GearboxTop_v3 (Autodesk Fusion 360 design; units mm, degrees)
Autodesk Fusion 360 part; units mm, degrees
sketch "Sketch1" plane through (0, 0, 0) normal (0, 0, 1) x (1, 0, 0)
  circle A0 centre (0, 0) radius 65
  circle A1 centre (0, 0) radius 61.0225 construction
  circle A2 centre (0, 0) radius 39.5
  circle A3 centre (0, -61.0225) radius 1.5
  dimension "d1" = 130
  dimension "d2" = 122.045
  dimension "d3" = 79
  dimension "ScrewDia" = 3
  constraint coincident A0.centre A1.centre
  constraint concentric A0 A1
  constraint coincident A1 A3.centre
  measures "d1" diameter of A0
  measures "d2" diameter of A1
  measures "d3" diameter of A2
  measures "ScrewDia" diameter of A3
extrude "Extrude1" add sketch "Sketch1" along normal blind 2 contours A0 | A3
sketch "Sketch2" plane through (0, 0, 2) normal (0, 0, 1) x (-1, 0, 0)
  circle A0 centre (0, 0) radius 39.5
  circle A1 centre (0, 0) radius 65
  circle A2 centre (0, 0) radius 42.5
  dimension "BearingDia" = 85
  constraint coincident A0.centre A1.centre
  measures "BearingDia" diameter of A2
extrude "Extrude2" add sketch "Sketch2" along normal blind 10 contours A1
extrude "Extrude3" cut sketch "Sketch1" along normal blind 25 contours A3
sketch "Sketch3" plane through (0, 0, 12) normal (0, 0, 1) x (-1, 0, 0)
  circle A0 centre (0, 61.0225) radius 1.5
  circle A1 centre (0, 0) radius 42.5
  circle A2 centre (0, 0) radius 65
  circle A3 centre (0, -61.0225) radius 2.5
  dimension "ScrewHeadDia" = 5
  measures "ScrewHeadDia" diameter of A3
extrude "Extrude4" cut sketch "Sketch3" against normal blind 3 contours A3
sketch "Sketch6" plane through (0, 0, 0) normal (0, 0, -1) x (1, 0, 0)
  circle A0 centre (0, 61.0225) radius 1.5
  circle A1 centre (0, 0) radius 39.5
  circle A2 centre (0, 0) radius 65
  circle A3 centre (0, 61.0225) radius 2.5
  dimension "d37" = 5
  constraint concentric A0 A3
  measures "d37" diameter of A3
extrude "Extrude6" cut sketch "Sketch6" against normal blind 3 contours A3
pattern_circular "C-Pattern1" count 6 over 360 about axis through (0, 0, 1.75) along (0, 0, 1) of "Extrude3", "Extrude4"
sketch "Sketch4" plane through (0, 0, 0) normal (0, 0, 1) x (1, 0, 0)
sketch "Sketch5" plane through (0, 0, 0) normal (0, 0, 1) x (1, 0, 0)
  line L0 (0, 5) -> (80, 5)
  line L1 (80, 5) -> (80, -5)
  line L2 (80, -5) -> (0, -5)
  line L3 (0, -5) -> (0, 5)
  line L4 (-4.3301, -2.5) -> (-44.3301, 66.782)
  line L5 (-35.6699, 71.782) -> (4.3301, 2.5)
  line L6 (-44.3301, 66.782) -> (-35.6699, 71.782)
  line L7 (4.3301, 2.5) -> (-4.3301, -2.5)
  line L8 (4.3301, -2.5) -> (-35.6699, -71.782)
  line L9 (-44.3301, -66.782) -> (-4.3301, 2.5)
  line L10 (-35.6699, -71.782) -> (-44.3301, -66.782)
  line L11 (-4.3301, 2.5) -> (4.3301, -2.5)
  circle A0 centre (0, 0) radius 65
  dimension "d17" = 80
  dimension "d18" = 10
  dimension "d19" = 5
  dimension "d21" = 360
  dimension "d22" = 130
  constraint horizontal L0
  constraint vertical L1
  constraint horizontal L2
  constraint vertical L3
  constraint coincident A0.centre origin
  measures "d17" distance of L0.start L0.end
  measures "d18" distance of L0.start L2.end
  measures "d19" distance of A0.centre L0.start
  measures "d22" diameter of A0
extrude "Extrude5" add sketch "Sketch5" along normal blind 12 contours L0 L1 L2 A0 | L4 L5 L6 A0 | L8 L9 L10 A0
fillet "Fillet1" radius 5 6 edges at (-36.7338, -53.6249, 6) (-36.7338, 53.6249, 6) (-28.0736, 58.6249, 6) (64.8074, 5, 6) (64.8074, -5, 6) (-28.0736, -58.6249, 6)
fillet "Fillet1" radius 2.5 9 edges at (-31.8717, 65.2034, 12) (-40, 69.282, 12) (-40.532, 60.2034, 12) (-40.532, -60.2034, 12) (-40, -69.282, 12) (-31.8717, -65.2034, 12) (72.4037, -5, 12) (72.4037, 5, 12) (80, 0, 12)
hole "Hole1" at (74.4188, 0.0203, 12) direction (0, 0, -1) diameter 3 end through all
hole "Hole2" at (74.4188, 0.0203, 12) direction (0, 0, -1) diameter 5 depth 5 tip angle 118
pattern_circular "C-Pattern2" count 3 over 360 about axis through (0, 0, 1.75) along (0, 0, 1) of "Hole1", "Hole2"
pattern_circular "C-Pattern3" count 6 over 360 about axis through (0, 0, 1.75) along (0, 0, 1) of "Extrude6"
equation "BearingHieght = 10 mm"
equation "ScrewHeadDepth = -3 mm"
